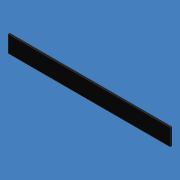
# Autodesk Inventor part: cRIO-FRC Pad
Saved by Autodesk Inventor 2011 (Build 150239000, 239)
## iProperties
Category: FRC Parts
Manager: Ed Sparks
Company: FirstCadLibrary
Shininess: 64.0
Length Units: 11272
Angle Units: 11279
Time Units: 11290
Mass Units: 11286
Length Display Precision: 3
Angle Display Precision: 2
Compacted: True
Part Number: cRIO-FRC Pad
Document SubType Name: Modeling
Created: 2008-12-13
Designer: Ed Sparks
Project: FIRST
Catalog Web Link: www.firstcadlibrary.com
Engineer: Ed Sparks
Material: ABS Plastic
Density: 1 g/cm^3
Density: 0.0
Volumn: 0.0
Area: 0.0
PropertySet Name: Model Information
Control State: 0
Master: False
Checked Out: False
Author: Ed Sparks
Keywords: FIRST
Autodesk Inventor part; units mm, degrees
ref_plane "YZ Plane" through (0, 0, 0) normal (1, 0, 0) x (0, 1, 0)
ref_plane "XZ Plane" through (0, 0, 0) normal (0, 1, 0) x (-1, 0, 0)
ref_plane "XY Plane" through (0, 0, 0) normal (0, 0, 1) x (1, 0, 0)
sketch "Sketch1" plane through (0, 0, 0) normal (0, 0, 1) x (1, 0, 0)
  line L0 (-92.075, 9.525) -> (92.075, 9.525)
  line L1 (92.075, 9.525) -> (92.075, -9.525)
  line L2 (92.075, -9.525) -> (-92.075, -9.525)
  line L3 (-92.075, -9.525) -> (-92.075, 9.525)
  line L4 (0, 0) -> (0, 9.525) construction
  line L5 (0, 0) -> (0, -9.525) construction
  line L6 (0, 0) -> (-92.075, 0) construction
  line L7 (0, 0) -> (92.075, 0) construction
  dimension "d0" = 184.15
  dimension "d1" = 19.05
  constraints: 16 end point, 4 midpoint, 2 collinear, 2 parallel, 1 horizontal, 1 perpendicular, 1 other
  measures "d0" distance of L0.start L0.end
  measures "d1" distance of L2.end L0.start
extrude "Extrusion1" add sketch "Sketch1" along normal mid plane 1.905
body "Solid1"
